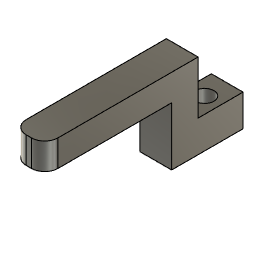
wire_clamp (Autodesk Fusion 360 design; units mm, degrees)
Autodesk Fusion 360 part; units mm, degrees
sketch "Sketch1" plane through (0, 0, 0) normal (0, 0, 1) x (1, 0, 0)
  circle A0 centre (0, 0) radius 1.75
  circle A1 centre (0, 0) radius 5
  circle A2 centre (0, 0) radius 3.5
  circle A3 centre (-26, 0) radius 4
  line L0 (-25.9137, 3.9991) -> (-3.0012, 3.9991)
  line L1 (-25.9137, -3.9991) -> (-3.0012, -3.9991)
  dimension "d1" = 3.5
  dimension "d2" = 10
  dimension "d3" = 7
  dimension "d4" = 8
  constraint coincident A0.centre A1.centre
  constraint concentric A1 A2
  constraint coincident A3 L0.start
  constraint coincident A1 L0.end
  constraint horizontal L0
  constraint coincident A3 L1.start
  constraint coincident A1 L1.end
  constraint parallel L0 L1
  measures "d1" diameter of A0
  measures "d2" diameter of A1
  measures "d3" diameter of A2
  measures "d4" diameter of A3
extrude "Extrude1" add sketch "Sketch1" against normal blind 18 contours A1 makes body 1
extrude "Extrude2" add sketch "Sketch1" along normal blind -12 and the other way blind 18 contours A2 bodies 1
extrude "Extrude3" add sketch "Sketch1" against normal blind 6 contours A1 A3 L0 L1 | A3 bodies 1
sketch "Sketch2" plane through (0, 0, 0) normal (1, 0, 0) x (0, 1, 0)
  line L0 (-10, 7) -> (14, 7)
  line L1 (14, 7) -> (14, 2)
  line L2 (14, 2) -> (-10, 2)
  line L3 (-10, 2) -> (-10, 7)
  line L4 (14, 7) -> (19, 7)
  line L5 (19, 7) -> (19, -9)
  line L6 (19, -9) -> (14, -9)
  line L7 (14, -9) -> (14, 7)
  line L8 (19, -9) -> (27.5, -9)
  line L9 (27.5, -9) -> (27.5, -3)
  line L10 (27.5, -3) -> (19, -3)
  line L11 (19, -3) -> (19, -9)
  constraint horizontal L0
  constraint vertical L1
  constraint horizontal L2
  constraint vertical L3
  constraint horizontal L4
  constraint vertical L5
  constraint horizontal L6
  constraint vertical L7
  constraint horizontal L8
  constraint vertical L9
  constraint horizontal L10
  constraint vertical L11
extrude "Extrude4" add sketch "Sketch2" against normal blind 6 separate body makes body 2
sketch "Sketch3" plane through (0, 0, -3) normal (0, 0, 1) x (-1, 0, 0)
  line L0 (0, -19) -> (0, -27.5)
  line L1 (0, -27.5) -> (6, -27.5)
  line L2 (6, -27.5) -> (6, -19)
  line L3 (6, -19) -> (0, -19)
  circle A0 centre (3, -23.25) radius 1.75
  dimension "d15" = 3.5
  measures "d15" diameter of A0
extrude "Extrude5" cut sketch "Sketch3" against normal blind 15 contours A0 bodies 2
fillet "Fillet1" radius 2.5 2 edges at (-6, -10, 4.5) (0, -10, 4.5) on bodies 2
hidden bodies 1
named bodies: "wire_clamp2", "wire_clamp1"
